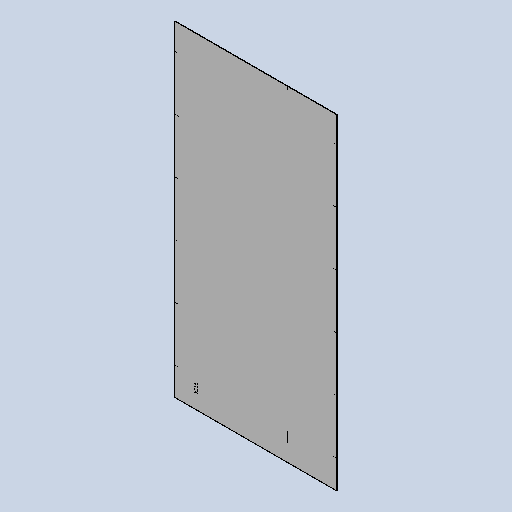
# Autodesk Inventor part: GBK 3328 shield 8
Saved by Autodesk Inventor 2026.2 (Build 302298010, 298A)
## iProperties
Created: 2026-04-17
Part Number: GBK 3328 shield 8
Material: Steel
Document SubType Name: Sheet Metal
Designer: pokla
Stock Number: 3328
Mass: 138487 g
Surface Area: 88564.8 cm^2
Volume: 17641.6 cm^3
Density: 7.85 g/cm^3
Sheet Metal Rule: Default_mm
Sheet Metal Width: 2980,000 mm
Sheet Metal Length: 1480,000 mm
Sheet Metal Area: 4410400,000 mm^2
Appearance: Default
Flat Pattern Width: 298 cm
Flat Pattern Length: 148 cm
Flat Pattern Area: 44104 cm^2
Author: admin
Autodesk Inventor part; units mm, degrees
ref_plane "YZ Plane" through (0, 0, 0) normal (1, 0, 0) x (0, 1, 0)
ref_plane "XZ Plane" through (0, 0, 0) normal (0, 1, 0) x (-1, 0, 0)
ref_plane "XY Plane" through (0, 0, 0) normal (0, 0, 1) x (1, 0, 0)
sketch "Sketch1" plane through (0, 0, 0) normal (0, 0, 1) x (1, 0, 0)
  line L0 (740, -1490) -> (-740, -1490)
  line L1 (-740, -1490) -> (-740, 1490)
  line L2 (-740, 1490) -> (740, 1490)
  line L3 (740, 1490) -> (740, -1490)
  line L4 (740, -1490) -> (-740, 1490) construction
  line L5 (-740, -1490) -> (740, 1490) construction
  point P0 (0, 0)
  dimension "d0" = 1480
  dimension "d1" = 2980
  measures "d0" distance of L1.end L2.end
  measures "d1" distance of L0.end L1.end
extrude "Plate1" add sketch "Sketch1" along normal blind 4
sketch "Эскиз3" plane through (0, 0, 0) normal (0, 0, -1) x (-1, 0, 0)
  line L0 (567.5874, -1279.3136) -> (567.5874, -1777.4498) construction
  line L1 (567.5874, -1777.4498) -> (527.9602, -1777.4498) construction
  line L2 (527.9602, -1777.4498) -> (527.9602, -1279.3136) construction
  line L3 (527.9602, -1279.3136) -> (567.5874, -1279.3136) construction
  line L4 (209.363, -1238) -> (209.363, -1335) projected
  line L5 (209.363, -1335) -> (205.363, -1335) projected
  line L6 (-290.5101, -1238) -> (-290.5101, -1335) projected
  line L7 (-290.5101, -1335) -> (-294.5101, -1335) projected
  line L8 (-290.5101, 1460.5) -> (-290.5101, 1520.5) projected
  line L9 (-290.5101, 1460.5) -> (-294.5101, 1460.5) projected
  line L10 (209.363, 1460.5) -> (209.363, 1520.5) projected
  line L11 (209.363, 1460.5) -> (205.363, 1460.5) projected
  line L12 (739.6246, -1234.5) -> (739.6246, -1230.5) projected
  line L13 (-740, -1234.5) -> (-710, -1234.5) projected
  line L14 (-710, -1234.5) -> (-710, -1230.5) projected
  line L15 (-740, -737.8333) -> (-710, -737.8333) projected
  line L16 (-710, -737.8333) -> (-710, -733.8333) projected
  line L17 (-740, -241.1667) -> (-710, -241.1667) projected
  line L18 (-710, -241.1667) -> (-710, -237.1667) projected
  line L19 (-740, 255.5) -> (-710, 255.5) projected
  line L20 (-710, 255.5) -> (-710, 259.5) projected
  line L21 (-740, 752.1667) -> (-710, 752.1667) projected
  line L22 (-710, 752.1667) -> (-710, 756.1667) projected
  line L23 (-740, 1248.8333) -> (-710, 1248.8333) projected
  line L24 (-710, 1248.8333) -> (-710, 1252.8333) projected
  line L25 (739.6246, -737.8333) -> (739.6246, -733.8333) projected
  line L26 (739.6246, -241.1667) -> (739.6246, -237.1667) projected
  line L27 (739.6246, 255.5) -> (739.6246, 259.5) projected
  line L28 (739.6246, 752.1667) -> (739.6246, 756.1667) projected
  line L29 (739.6246, 1248.8333) -> (739.6246, 1252.8333) projected
  line L30 (739.6246, 1248.8333) -> (709.6246, 1248.8333)
  line L31 (739.6246, 752.1667) -> (709.6246, 752.1667)
  line L32 (739.6246, 255.5) -> (709.6246, 255.5)
  line L33 (739.6246, -241.1667) -> (709.6246, -241.1667)
  line L34 (739.6246, -737.8333) -> (709.6246, -737.8333)
  line L35 (739.6246, -1234.5) -> (709.6246, -1234.5)
  point P0 (0, 0)
  dimension "d12" = 30
  dimension "d13" = 30
  dimension "d14" = 30
  dimension "d15" = 30
  dimension "d16" = 30
  dimension "d17" = 30
  constraints: 12 end point, 6 horizontal, 2 other
  measures "d12" distance of L29.start L30.end
  measures "d13" distance of L31.start L31.end
  measures "d14" distance of L32.start L32.end
  measures "d15" distance of L33.start L33.end
  measures "d16" distance of L34.start L34.end
  measures "d17" distance of L35.start L35.end
mark "Маркировка2"
equation "\"d0\" = Лист_ширина"
equation "\"d2\" = Thickness"
equation "\"BendRadius\" = Thickness"
equation "\"BendReliefWidth\" = Thickness"
equation "\"BendReliefDepth\" = 0.5 * Thickness"
equation "\"CornerReliefSize\" = 4 * Thickness"
equation "\"MinimumRemnant\" = 2 * Thickness"
equation "\"TransitionRadius\" = BendRadius"
equation "\"JacobiRadiusSize\" = BendRadius"
equation "\"GapSize\" = Thickness"
equation "\"Лист_ширина\" = 1480"
equation "\"Thickness\" = 4"
body "Solid1"
